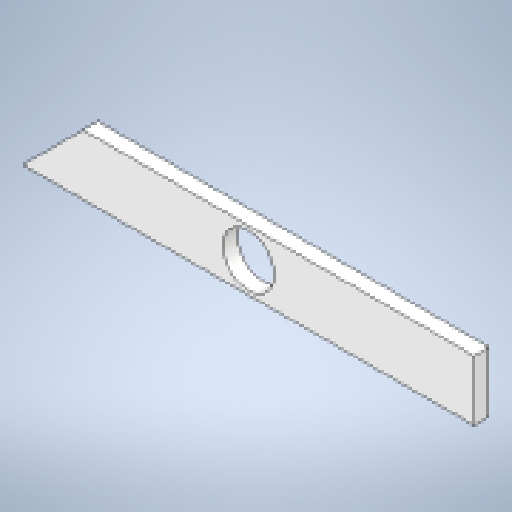
# Autodesk Inventor part: Side_Plate
Saved by Autodesk Inventor 2023.2 (Build 272271000, 271)
## iProperties
Created: 2024-01-26
Part Number: Side_Plate
Material: UHMW, White
Document SubType Name: Modeling
Designer: Nathan Cai
Density: 0.94 g/cm^3
Appearance: Smooth - White
Mass: 24.6877 g
Surface Area: 113.583 cm^2
Volume: 26.2635 cm^3
Author: Nathan Cai
Autodesk Inventor part; units mm, degrees
ref_plane "YZ Plane" through (0, 0, 0) normal (1, 0, 0) x (0, 1, 0)
ref_plane "XZ Plane" through (0, 0, 0) normal (0, 1, 0) x (-1, 0, 0)
ref_plane "XY Plane" through (0, 0, 0) normal (0, 0, 1) x (1, 0, 0)
sketch "Sketch1" plane through (0, 0, 0) normal (0, 0, 1) x (1, 0, 0)
  line L0 (0, 0) -> (190.5, 0)
  line L1 (190.5, 0) -> (190.5, 25.4)
  line L2 (190.5, 25.4) -> (0, 25.4)
  line L3 (0, 25.4) -> (0, 0)
  line L4 (0, 12.7) -> (190.5, 12.7) construction
  circle A0 centre (95.25, 12.7) radius 11
  line L5 (0, 0) -> (25.4, 25.4)
  circle A1 centre (177.8, 15.875) radius 25.4 construction
  circle A2 centre (177.8, 15.875) radius 1.7526
  circle A3 centre (44.45, 9.525) radius 1.7526
  dimension "d0" = 190.5
  dimension "d1" = 25.4
  dimension "d6" = 22
  dimension "d7" = 95.25
  dimension "d8" = 45
  dimension "d9" = 50.8
  dimension "d10" = 3.5052
  dimension "d11" = 12.7
  dimension "d12" = 9.525
  dimension "d13" = 3.5052
  dimension "d14" = 9.525
  dimension "d15" = 44.45
  constraints: 12 end point, 4 centre point, 3 midpoint, 2 parallel, 1 coincident, 1 horizontal, 1 perpendicular, 1 point on line
  measures "d0" distance of L2.end L1.end
  measures "d1" distance of L1.end L0.end
  measures "d6" diameter of A0
  measures "d7" distance from line of L1 A0.centre
  measures "d8" angle of L0 L5
  measures "d9" diameter of A1
  measures "d10" diameter of A2
  measures "d11" distance from line of L1 A2.centre
  measures "d12" distance from line of L2 A2.centre
  measures "d13" diameter of A3
  measures "d14" distance from line of L0 A3.centre
  measures "d15" distance from line of L3 A3.centre
extrude "Extrusion1" add sketch "Sketch1" along normal blind 6.35 contours L5 L2 L1 L0
body "Solid1"
